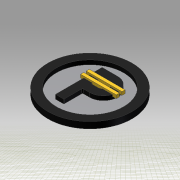
# Autodesk Inventor part: PennyKoin-3D-Inventor
Saved by Autodesk Inventor 2012 SP2 (Build 160219200, 219)
## iProperties
Created: 2018-12-19
Part Number: PennyKoin-3D-Inventor
Material: Default
Document SubType Name: Modeling
Designer: alesb
Density: 1 g/cm^3
Mass: 785.398 g
Surface Area: 785.398 cm^2
Volume: 785.398 cm^3
Author: alesb
Autodesk Inventor part; units mm, degrees
ref_plane "YZ Plane" through (0, 0, 0) normal (1, 0, 0) x (0, 1, 0)
ref_plane "XZ Plane" through (0, 0, 0) normal (0, 1, 0) x (-1, 0, 0)
ref_plane "XY Plane" through (0, 0, 0) normal (0, 0, 1) x (1, 0, 0)
sketch "Sketch1" plane through (0, 0, 0) normal (0, 0, 1) x (1, 0, 0)
  circle A0 centre (0, 0) radius 100
  circle A1 centre (0, 0) radius 80
  line L0 (-26.6667, -55.5556) -> (-26.6667, 55.5556)
  line L1 (-26.6667, 55.5556) -> (10, 55.5556)
  arc A2 (10, -11.1111) -> (10, 55.5556) centre (10, 22.2222) ccw
  line L2 (10, -11.1111) -> (-6.6667, -11.1111)
  line L3 (-6.6667, -11.1111) -> (-6.6667, -55.5556)
  line L4 (-6.6667, -55.5556) -> (-26.6667, -55.5556)
  line L5 (-6.6667, 35.5556) -> (10, 35.5556)
  arc A3 (10, 8.8889) -> (10, 35.5556) centre (10, 22.2222) ccw
  line L6 (10, 8.8889) -> (-6.6667, 8.8889)
  line L7 (-6.6667, 8.8889) -> (-6.6667, 35.5556)
  line L8 (-34.0741, 11.8519) -> (50.7407, 11.8519)
  line L9 (50.7407, 11.8519) -> (50.7407, 19.2593)
  line L10 (50.7407, 19.2593) -> (-34.0741, 19.2593)
  line L11 (-34.0741, 19.2593) -> (-34.0741, 11.8519)
  line L12 (-34.0741, 25.1852) -> (50.7407, 25.1852)
  line L13 (50.7407, 25.1852) -> (50.7407, 32.5926)
  line L14 (50.7407, 32.5926) -> (-34.0741, 32.5926)
  line L15 (-34.0741, 32.5926) -> (-34.0741, 25.1852)
  line L16 (1.6667, 8.8889) -> (1.6667, 32.5926) construction
  line L17 (1.6667, 35.5556) -> (1.6667, 11.8519) construction
  line L18 (0, 80) -> (0, 55.5556) construction
  line L19 (0, -80) -> (0, -11.1111) construction
  line L20 (-26.6667, 0) -> (0, 0) construction
  line L21 (50.7407, 25.1852) -> (50.7407, 19.2593) construction
  line L22 (50.7407, 22.2222) -> (10, 22.2222) construction
  line L23 (43.3333, 22.2222) -> (50.7407, 22.2222) construction
  point P0 (0, -45.5556)
  dimension "d0" = 20
  dimension "d1" = 200
  dimension "d2" = 20
  dimension "d3" = 20
  dimension "d4" = 7.4074
  dimension "d5" = 111.1111
  dimension "d6" = 2.963
  dimension "d7" = 7.4074
  dimension "d12" = 7.4074
  dimension "d50" = 44.4444
  dimension "d52" = 10
  dimension "d53" = 30
  constraints: 48 end point, 11 perpendicular, 9 parallel, 7 point on circle, 5 midpoint, 5 point on line, 4 centre point, 4 coincident, 4 collinear, 4 tangent, 3 equal length, 2 horizontal, 1 vertical, 1 vertical alignment
  measures "d0" radial gap between concentric circles of A0 A1
  measures "d1" diameter of A0
  measures "d2" distance between parallel lines of L0 L7
  measures "d3" radial gap between concentric circles of A2 A3
  measures "d4" distance between parallel lines of L0 L11
  measures "d5" distance of L0.start L0.end
  measures "d6" distance between parallel lines of L5 L14
  measures "d7" distance of L23.start L22.start
  measures "d12" distance between parallel lines of L12 L14
  measures "d50" distance of L2.end L3.end
  measures "d52" horizontal distance of L22.end point (0, 0)
extrude "Extrusion1" add sketch "Sketch1" along normal blind 10 contours A0 | L0 L8 L7 L6 A3 A2 L2 L3 L4 | L0 L10 L7 L8 | L0 L12 L7 L10 | L0 L14 L7 L12 | A3 L10 A2 L8 | L0 L1 A2 L14 A3 L5 L7 | A3 L12 A2 L10 | A3 L14 A2 L12
sketch "Sketch2" plane through (0, 0, 10) normal (0, 0, 1) x (1, 0, 0)
  line L0 (-34.0741, 25.1852) -> (50.7407, 25.1852) projected
  line L1 (50.7407, 32.5926) -> (-34.0741, 32.5926) projected
  line L2 (50.7407, 25.1852) -> (50.7407, 32.5926) projected
  line L3 (-34.0741, 32.5926) -> (-34.0741, 25.1852) projected
  line L4 (50.7407, 19.2593) -> (-34.0741, 19.2593) projected
  line L5 (-34.0741, 19.2593) -> (-34.0741, 11.8519) projected
  line L6 (-34.0741, 11.8519) -> (50.7407, 11.8519) projected
  line L7 (50.7407, 11.8519) -> (50.7407, 19.2593) projected
  point P0 (0, 0)
extrude "Extrusion2" add sketch "Sketch2" against normal blind 4
sketch "Sketch3" plane through (0, 0, 0) normal (0, 0, -1) x (-1, 0, 0)
  circle A0 centre (0, 0) radius 100 projected
extrude "Extrusion3" add sketch "Sketch3" along normal blind 5
fillet "Fillet2" radius 2 2 edges at (-6.6667, 8.8889, 5) (-6.6667, 35.5556, 5)
fillet "Fillet3" radius 2 1 edges at (-6.6667, -11.1111, 5)
chamfer "Chamfer1" distance 0.5 angle 45 3 edges at (-26.6667, 55.5556, 5) (-26.6667, -55.5556, 5) (-6.6667, -55.5556, 5)
sketch "Sketch6" plane through (0, 0, 10) normal (0, 0, 1) x (1, 0, 0)
  line L0 (50.7407, 32.5926) -> (-34.0741, 32.5926)
  line L1 (-34.0741, 32.5926) -> (-34.0741, 25.1852)
  line L2 (-34.0741, 25.1852) -> (50.7407, 25.1852)
  line L3 (50.7407, 25.1852) -> (50.7407, 32.5926)
  line L4 (-34.0741, 19.2593) -> (50.7407, 19.2593)
  line L5 (50.7407, 19.2593) -> (50.7407, 11.8519)
  line L6 (50.7407, 11.8519) -> (-34.0741, 11.8519)
  line L7 (-34.0741, 11.8519) -> (-34.0741, 19.2593)
  point P0 (0, 0)
  constraints: 16 end point, 4 parallel, 2 horizontal, 2 perpendicular
extrude "Extrusion5" add sketch "Sketch6" along normal blind 4
equation "\"d0\" = 0.1 * d1"
equation "\"d2\" = d0"
equation "\"d3\" = d2"
equation "\"d4\" = 0.0666667 * d5"
equation "\"d5\" = 0.555556 * d1"
equation "\"d6\" = 0.4 * d4"
equation "\"d7\" = d4"
equation "\"d12\" = d4"
equation "\"d50\" = 0.4 * d5"
equation "\"d52\" = 0.5 * d0"
equation "\"d53\" = 3 * d52"
body "Solid1"
